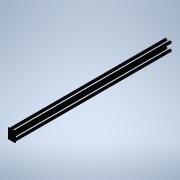
# Autodesk Inventor part: 1000
Saved by Autodesk Inventor 2020 (Build 240168000, 168)
## iProperties
Created: 2020-07-08
Part Number: 1000
Material: Generic
Document SubType Name: Modeling
Designer: Vikki
Density: 1 g/cm^3
Appearance: Anodized - Black
Mass: 1325.96 g
Surface Area: 11888.6 cm^2
Volume: 1325.96 cm^3
Author: Vikki
Autodesk Inventor part; units mm, degrees
ref_plane "YZ Plane" through (0, 0, 0) normal (1, 0, 0) x (0, 1, 0)
ref_plane "XZ Plane" through (0, 0, 0) normal (0, 1, 0) x (-1, 0, 0)
ref_plane "XY Plane" through (0, 0, 0) normal (0, 0, 1) x (1, 0, 0)
sketch "Sketch1" plane through (0, 0, 0) normal (0, 0, 1) x (1, 0, 0)
  line L0 (3.1, 9.8) -> (3.1, 8.2) projected
  arc A0 (3.1, 8.2) -> (3.3, 8) centre (3.3, 8.2) ccw projected
  line L1 (3.3, 8) -> (6.1029, 8) projected
  arc A1 (6.2444, 7.6586) -> (6.1029, 8) centre (6.1029, 7.8) ccw projected
  line L2 (6.2444, 7.6586) -> (2.6444, 4.0586) projected
  arc A2 (2.5029, 4) -> (2.6444, 4.0586) centre (2.5029, 4.2) ccw projected
  line L3 (2.5029, 4) -> (-2.5029, 4) projected
  arc A3 (-2.6444, 4.0586) -> (-2.5029, 4) centre (-2.5029, 4.2) ccw projected
  line L4 (-2.6444, 4.0586) -> (-6.2444, 7.6586) projected
  arc A4 (-6.1029, 8) -> (-6.2444, 7.6586) centre (-6.1029, 7.8) ccw projected
  line L5 (-6.1029, 8) -> (-3.3, 8) projected
  arc A5 (-3.3, 8) -> (-3.1, 8.2) centre (-3.3, 8.2) ccw projected
  line L6 (-3.1, 8.2) -> (-3.1, 9.8) projected
  arc A6 (-3.1, 9.8) -> (-3.3, 10) centre (-3.3, 9.8) ccw projected
  line L7 (-3.3, 10) -> (-8.5, 10) projected
  arc A7 (-8.5, 10) -> (-10, 8.5) centre (-8.5, 8.5) ccw projected
  line L8 (-10, 8.5) -> (-10, 3.3) projected
  arc A8 (-10, 3.3) -> (-9.8, 3.1) centre (-9.8, 3.3) ccw projected
  line L9 (-9.8, 3.1) -> (-8.2, 3.1) projected
  arc A9 (-8.2, 3.1) -> (-8, 3.3) centre (-8.2, 3.3) ccw projected
  line L10 (-8, 3.3) -> (-8, 6.1029) projected
  arc A10 (-7.6586, 6.2444) -> (-8, 6.1029) centre (-7.8, 6.1029) ccw projected
  line L11 (-7.6586, 6.2444) -> (-4.0586, 2.6444) projected
  arc A11 (-4, 2.5029) -> (-4.0586, 2.6444) centre (-4.2, 2.5029) ccw projected
  line L12 (-4, 2.5029) -> (-4, -2.5029) projected
  arc A12 (-4.0586, -2.6444) -> (-4, -2.5029) centre (-4.2, -2.5029) ccw projected
  line L13 (-4.0586, -2.6444) -> (-7.6586, -6.2444) projected
  arc A13 (-8, -6.1029) -> (-7.6586, -6.2444) centre (-7.8, -6.1029) ccw projected
  line L14 (-8, -6.1029) -> (-8, -3.3) projected
  arc A14 (-8, -3.3) -> (-8.2, -3.1) centre (-8.2, -3.3) ccw projected
  line L15 (-8.2, -3.1) -> (-9.8, -3.1) projected
  arc A15 (-9.8, -3.1) -> (-10, -3.3) centre (-9.8, -3.3) ccw projected
  line L16 (-10, -3.3) -> (-10, -8.5) projected
  arc A16 (-10, -8.5) -> (-8.5, -10) centre (-8.5, -8.5) ccw projected
  line L17 (-8.5, -10) -> (-3.3, -10) projected
  arc A17 (-3.3, -10) -> (-3.1, -9.8) centre (-3.3, -9.8) ccw projected
  line L18 (-3.1, -9.8) -> (-3.1, -8.2) projected
  arc A18 (-3.1, -8.2) -> (-3.3, -8) centre (-3.3, -8.2) ccw projected
  line L19 (-3.3, -8) -> (-6.1029, -8) projected
  arc A19 (-6.2444, -7.6586) -> (-6.1029, -8) centre (-6.1029, -7.8) ccw projected
  line L20 (-6.2444, -7.6586) -> (-2.6444, -4.0586) projected
  arc A20 (-2.5029, -4) -> (-2.6444, -4.0586) centre (-2.5029, -4.2) ccw projected
  line L21 (-2.5029, -4) -> (2.5029, -4) projected
  arc A21 (2.6444, -4.0586) -> (2.5029, -4) centre (2.5029, -4.2) ccw projected
  line L22 (2.6444, -4.0586) -> (6.2444, -7.6586) projected
  arc A22 (6.1029, -8) -> (6.2444, -7.6586) centre (6.1029, -7.8) ccw projected
  line L23 (6.1029, -8) -> (3.3, -8) projected
  arc A23 (3.3, -8) -> (3.1, -8.2) centre (3.3, -8.2) ccw projected
  line L24 (3.1, -8.2) -> (3.1, -9.8) projected
  arc A24 (3.1, -9.8) -> (3.3, -10) centre (3.3, -9.8) ccw projected
  line L25 (3.3, -10) -> (8.5, -10) projected
  arc A25 (8.5, -10) -> (10, -8.5) centre (8.5, -8.5) ccw projected
  line L26 (10, -8.5) -> (10, -3.3) projected
  arc A26 (10, -3.3) -> (9.8, -3.1) centre (9.8, -3.3) ccw projected
  line L27 (9.8, -3.1) -> (8.2, -3.1) projected
  arc A27 (8.2, -3.1) -> (8, -3.3) centre (8.2, -3.3) ccw projected
  line L28 (8, -3.3) -> (8, -6.1029) projected
  arc A28 (7.6586, -6.2444) -> (8, -6.1029) centre (7.8, -6.1029) ccw projected
  line L29 (7.6586, -6.2444) -> (4.0586, -2.6444) projected
  arc A29 (4, -2.5029) -> (4.0586, -2.6444) centre (4.2, -2.5029) ccw projected
  line L30 (4, -2.5029) -> (4, 2.5029) projected
  arc A30 (4.0586, 2.6444) -> (4, 2.5029) centre (4.2, 2.5029) ccw projected
  line L31 (4.0586, 2.6444) -> (7.6586, 6.2444) projected
  arc A31 (8, 6.1029) -> (7.6586, 6.2444) centre (7.8, 6.1029) ccw projected
  line L32 (8, 6.1029) -> (8, 3.3) projected
  arc A32 (8, 3.3) -> (8.2, 3.1) centre (8.2, 3.3) ccw projected
  line L33 (8.2, 3.1) -> (9.8, 3.1) projected
  arc A33 (9.8, 3.1) -> (10, 3.3) centre (9.8, 3.3) ccw projected
  line L34 (10, 3.3) -> (10, 8.5) projected
  arc A34 (10, 8.5) -> (8.5, 10) centre (8.5, 8.5) ccw projected
  line L35 (8.5, 10) -> (3.3, 10) projected
  arc A35 (3.3, 10) -> (3.1, 9.8) centre (3.3, 9.8) ccw projected
  circle A36 centre (0, 0) radius 2 projected
extrude "Extrusion1" add sketch "Sketch1" along normal blind 1750
pattern_linear "Rectangular Pattern1" count 2 spacing 80 along (0, 1, 0) of "Extrusion1"
pattern_linear "Rectangular Pattern2" count 2 spacing 50 along (1, 0, 0) of "Extrusion1", "Rectangular Pattern1"
sketch "Sketch3" plane through (41.5, 10, 1750) normal (0, 0, 1) x (1, 0, 0)
  point P0 (-41.5, -10)
body "Solid1"
